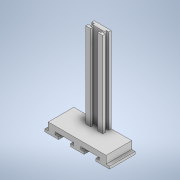
# Autodesk Inventor part: Clamp jaw handle
Saved by Autodesk Inventor 2022 (Build 260153000, 153)
## iProperties
Created: 2021-06-24
Part Number: Clamp jaw handle
Material: Generic
Document SubType Name: Modeling
Designer: Admin
Density: 1 g/cm^3
Appearance: Default
Author: Admin
Autodesk Inventor part; units mm, degrees
ref_plane "YZ Plane" through (0, 0, 0) normal (1, 0, 0) x (0, 1, 0)
ref_plane "XZ Plane" through (0, 0, 0) normal (0, 1, 0) x (-1, 0, 0)
ref_plane "XY Plane" through (0, 0, 0) normal (0, 0, 1) x (1, 0, 0)
sketch "Sketch1" plane through (0, 0, 0) normal (0, 0, 1) x (1, 0, 0)
  line L0 (-300, 0) -> (300, 0)
  line L1 (300, 0) -> (300, 50)
  line L2 (-300, 50) -> (-300, 0)
  line L3 (-20, 50) -> (-20, 35)
  line L4 (-20, 35) -> (-40, 35)
  line L5 (-40, 35) -> (-40, 20)
  line L6 (-40, 20) -> (40, 20)
  line L7 (40, 20) -> (40, 35)
  line L8 (40, 35) -> (20, 35)
  line L9 (20, 35) -> (20, 50)
  line L10 (-75, 159.793) -> (-75, -97.8722) construction
  line L11 (75, 159.793) -> (75, -92.8199) construction
  line L12 (-110, 20) -> (-190, 20)
  line L13 (-190, 20) -> (-190, 35)
  line L14 (-110, 35) -> (-110, 20)
  line L15 (-130, 35) -> (-110, 35)
  line L16 (-130, 50) -> (-130, 35)
  line L17 (-170, 35) -> (-170, 50)
  line L18 (-190, 35) -> (-170, 35)
  line L19 (170, 50) -> (170, 35)
  line L20 (170, 35) -> (190, 35)
  line L21 (190, 35) -> (190, 20)
  line L22 (190, 20) -> (110, 20)
  line L23 (110, 20) -> (110, 35)
  line L24 (110, 35) -> (130, 35)
  line L25 (130, 35) -> (130, 50)
  line L26 (-20, 50) -> (-130, 50)
  line L27 (-170, 50) -> (-300, 50)
  line L28 (300, 50) -> (170, 50)
  line L29 (130, 50) -> (20, 50)
  line L30 (170, 35) -> (170, 80)
  line L31 (170, 80) -> (-170, 80)
  line L32 (-170, 80) -> (-170, 35)
  point P0 (0, 0)
  point P1 (0, 0)
  dimension "d0" = 300
  dimension "d1" = 600
  dimension "d2" = 50
  dimension "d3" = 50
  dimension "d4" = 20
  dimension "d5" = 20
  dimension "d6" = 20
  dimension "d7" = 20
  dimension "d8" = 30
  dimension "d9" = 15
  dimension "d10" = 15
  dimension "d11" = 75
  dimension "d12" = 75
  dimension "d13" = 15
  dimension "d14" = 109.793
  dimension "d15" = 142.8199
  dimension "d16" = 109.793
  dimension "d17" = 147.8722
  dimension "d18" = 45
  constraints: 66 end point, 16 symmetric about line, 10 perpendicular, 5 parallel, 4 vertical, 2 horizontal, 1 point on line
  measures "d0" distance of point (0, 0) L0.start
  measures "d1" distance of L0.start L1.start
  measures "d2" distance of L2.start L0.start
  measures "d3" vertical distance of point (0, 0) L2.start
  measures "d4" horizontal distance of point (0, 0) L3.start
  measures "d5" horizontal distance of point (0, 0) L29.end
  measures "d6" distance of L3.end L4.end
  measures "d7" distance of L8.start L9.start
  measures "d8" vertical distance of L3.start L6.start
  measures "d9" distance of L4.end L6.start
  measures "d10" distance of L9.start L29.end
  measures "d11" distance from line of point (0, 0) L11
  measures "d12" distance from line of point (0, 0) L10
  measures "d13" distance between parallel lines of L24 L28
  measures "d14" distance from line of L11.start L28
  measures "d15" distance from line of L11.end L28
  measures "d16" distance from line of L10.start L28
  measures "d17" distance from line of L10.end L28
  measures "d18" distance of L19.end L30.end
sketch "Sketch2" plane through (0, 0, 0) normal (0, 0, 1) x (1, 0, 0)
  point P0 (0, 0)
extrude "Extrusion1" add sketch "Sketch1" along normal blind 150 contours L32 L31 L30 L19 L20 L21 L22 L23 L24 L25 L29 L9 L8 L7 L6 L5 L4 L3 L26 L16 L15 L14 L12 L13 L18 L17
sketch "Sketch3" plane through (-170, 80, 0) normal (0, 1, 0) x (1, 0, 0)
  line L0 (170, 0) -> (130, 0)
  line L1 (130, 0) -> (130, -50) construction
  line L2 (130, -50) -> (170, -50)
  line L3 (340, 0) -> (0, 0) projected
  line L4 (170, -50) -> (210, -50)
  line L5 (210, -50) -> (210, 0) construction
  line L6 (210, 0) -> (170, 0)
  line L7 (120, -50) -> (220, -50)
  line L8 (220, -50) -> (220, 0)
  line L9 (220, 0) -> (120, 0)
  line L10 (120, 0) -> (120, -50)
  line L11 (120, -50) -> (220, 0) construction
  line L12 (220, -50) -> (120, 0) construction
  point P0 (170, -25)
  dimension "d21" = 40
  dimension "d22" = 50
  dimension "d23" = 40
  dimension "d36" = 100
  constraints: 24 end point, 4 parallel, 3 horizontal, 3 perpendicular, 2 midpoint, 2 point on line
  measures "d21" distance of L2.end L1.end
  measures "d22" distance of L1.end L0.end
  measures "d23" distance of L6.end L5.end
  measures "d36" distance of L9.end L8.end
extrude "Extrusion2" add sketch "Sketch3" along normal blind 500
sketch "Sketch5" plane through (-170, 580, 0) normal (0, 1, 0) x (1, 0, 0)
  line L0 (150, 0) -> (150, -150) projected
  line L1 (190, -60) -> (150, -60)
  line L2 (150, -60) -> (150, -40)
  line L3 (150, -40) -> (190, -40) construction
  line L4 (190, -40) -> (190, -60)
  line L5 (220, -50) -> (120, -50) projected
  line L6 (190, -60) -> (150, -40) construction
  line L7 (150, -60) -> (190, -40) construction
  line L8 (150, -40) -> (140, -40)
  line L9 (140, -40) -> (140, -25)
  line L10 (140, -25) -> (200, -25)
  line L11 (200, -25) -> (200, -40)
  line L12 (200, -40) -> (190, -40)
  point P0 (170, 0)
  point P1 (170, -50)
  point P2 (210, -50)
  point P3 (130, -50)
  point P4 (170, -50)
  dimension "d26" = 10
  dimension "d27" = 15
  dimension "d28" = 60
  dimension "d31" = 20
  constraints: 22 end point, 5 perpendicular, 4 midpoint, 2 horizontal, 2 parallel, 2 point on line, 1 other
  measures "d26" distance of L2.end L8.end
  measures "d27" distance of L8.end L9.end
  measures "d28" distance of L9.end L10.end
  measures "d31" distance of L3.end L1.start
extrude "Extrusion3" cut sketch "Sketch5" against normal blind 500
sketch "Sketch6" plane through (-170, 580, 0) normal (0, 1, 0) x (1, 0, 0)
  line L0 (130, 0) -> (130, -150) projected
  line L1 (150, 0) -> (150, -150) projected
  line L2 (135, -30) -> (135, -20)
  line L3 (170, 0) -> (170, -54.7641) construction
  line L4 (120, -50) -> (120, 0) projected
  line L5 (120, -20) -> (120, -30)
  line L6 (220, 0) -> (220, -50) projected
  line L7 (135, -20) -> (135, -15)
  line L8 (135, -15) -> (120, -15)
  line L9 (120, -30) -> (120, -35)
  line L10 (120, -35) -> (135, -35)
  line L11 (135, -35) -> (135, -30)
  line L12 (120, -15) -> (120, -20)
  line L13 (205, -30) -> (205, -20)
  line L14 (220, -50) -> (220, 0)
  line L15 (205, -20) -> (205, -15)
  line L16 (205, -15) -> (220, -15)
  line L17 (220, -30) -> (220, -35)
  line L18 (220, -35) -> (205, -35)
  line L19 (205, -35) -> (205, -30)
  point P0 (130, -35)
  point P1 (130, -15)
  dimension "d38" = 5
  dimension "d39" = 15
  constraints: 32 end point, 8 point on line, 7 symmetric about line, 3 perpendicular, 2 vertical, 1 collinear
  measures "d38" distance of L5.end L9.end
  measures "d39" distance of L7.end L8.end
extrude "Extrusion4" cut sketch "Sketch6" against normal blind 500
body "Solid1"
